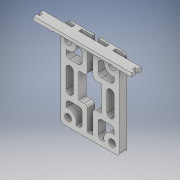
# Autodesk Inventor part: LED Riser
Saved by Autodesk Inventor 2017.3 (Build 213256000, 256)
## iProperties
Created: 2019-07-16
Part Number: LED Riser
Material: Generic
Document SubType Name: Modeling
Designer: LSabe
Density: 1 g/cm^3
Appearance: Default
Author: LSabe
Autodesk Inventor part; units mm, degrees
ref_plane "YZ Plane" through (0, 0, 0) normal (1, 0, 0) x (0, 1, 0)
ref_plane "XZ Plane" through (0, 0, 0) normal (0, 1, 0) x (-1, 0, 0)
ref_plane "XY Plane" through (0, 0, 0) normal (0, 0, 1) x (1, 0, 0)
sketch "Sketch1" plane through (0, 0, 0) normal (0, 0, 1) x (1, 0, 0)
  line L0 (-3.81, -7.6835) -> (45.466, -7.6835)
  line L1 (48.641, -4.5085) -> (48.641, 70.4215)
  line L2 (48.641, 70.4215) -> (-6.985, 70.4215)
  line L3 (-6.985, 70.4215) -> (-6.985, -4.5085)
  arc A0 (45.466, -7.6835) -> (48.641, -4.5085) centre (45.466, -4.5085) ccw
  arc A1 (-6.985, -4.5085) -> (-3.81, -7.6835) centre (-3.81, -4.5085) ccw
  line L4 (31.623, 19.304) -> (31.623, 43.434)
  line L5 (10.033, 43.434) -> (10.033, 19.304)
  line L6 (18.288, -7.6835) -> (23.368, -7.6835)
  line L7 (23.368, 70.4215) -> (18.288, 70.4215)
  arc A2 (-1.905, 55.0979) -> (7.874, 62.738) centre (0, 62.738) ccw
  arc A3 (33.782, 62.738) -> (43.561, 55.0979) centre (41.656, 62.738) ccw
  arc A4 (43.561, 7.6401) -> (34.2249, -2.6035) centre (41.656, 0) ccw
  arc A5 (7.4311, -2.6035) -> (-1.905, 7.6401) centre (0, 0) ccw
  line L8 (34.2249, -2.6035) -> (31.623, -2.6035)
  line L9 (10.033, -2.6035) -> (7.4311, -2.6035)
  line L10 (31.623, 43.434) -> (26.543, 43.434)
  line L11 (15.113, 43.434) -> (10.033, 43.434)
  line L12 (10.033, 19.304) -> (15.113, 19.304)
  line L13 (26.543, 19.304) -> (31.623, 19.304)
  line L14 (23.368, 46.609) -> (23.368, 62.738)
  line L15 (18.288, 62.738) -> (18.288, 46.609)
  line L16 (23.368, -2.6035) -> (23.368, 16.129)
  line L17 (18.288, 16.129) -> (18.288, -2.6035)
  line L18 (18.288, -2.6035) -> (23.368, -2.6035)
  line L19 (28.448, 51.689) -> (28.448, 59.563)
  line L20 (40.386, 48.514) -> (31.623, 48.514)
  line L21 (13.208, 59.563) -> (13.208, 51.689)
  line L22 (10.033, 48.514) -> (1.27, 48.514)
  line L23 (13.208, 11.049) -> (13.208, 0.5715)
  line L24 (1.27, 14.224) -> (10.033, 14.224)
  line L25 (31.623, 14.224) -> (40.386, 14.224)
  line L26 (28.448, 0.5715) -> (28.448, 11.049)
  line L27 (-1.905, 7.6401) -> (-1.905, 11.049)
  line L28 (-1.905, 51.689) -> (-1.905, 55.0979)
  line L29 (43.561, 55.0979) -> (43.561, 51.689)
  line L30 (43.561, 11.049) -> (43.561, 7.6401)
  line L31 (43.561, 22.479) -> (43.561, 40.259)
  line L32 (-1.905, 40.259) -> (-1.905, 22.479)
  line L33 (4.953, 40.259) -> (4.953, 22.479)
  line L34 (36.703, 22.479) -> (36.703, 40.259)
  line L35 (1.27, 43.434) -> (1.778, 43.434)
  line L36 (1.778, 19.304) -> (1.27, 19.304)
  line L37 (39.878, 43.434) -> (40.386, 43.434)
  line L38 (40.386, 19.304) -> (39.878, 19.304)
  arc A6 (10.033, 48.514) -> (13.208, 51.689) centre (10.033, 51.689) ccw
  arc A7 (28.448, 51.689) -> (31.623, 48.514) centre (31.623, 51.689) ccw
  arc A8 (31.623, 14.224) -> (28.448, 11.049) centre (31.623, 11.049) ccw
  arc A9 (13.208, 11.049) -> (10.033, 14.224) centre (10.033, 11.049) ccw
  arc A10 (1.27, 14.224) -> (-1.905, 11.049) centre (1.27, 11.049) ccw
  arc A11 (10.033, -2.6035) -> (13.208, 0.5715) centre (10.033, 0.5715) ccw
  arc A12 (28.448, 0.5715) -> (31.623, -2.6035) centre (31.623, 0.5715) ccw
  arc A13 (43.561, 11.049) -> (40.386, 14.224) centre (40.386, 11.049) ccw
  arc A14 (40.386, 48.514) -> (43.561, 51.689) centre (40.386, 51.689) ccw
  arc A15 (-1.905, 51.689) -> (1.27, 48.514) centre (1.27, 51.689) ccw
  arc A16 (23.368, 46.609) -> (26.543, 43.434) centre (26.543, 46.609) ccw
  arc A17 (15.113, 43.434) -> (18.288, 46.609) centre (15.113, 46.609) ccw
  arc A18 (18.288, 16.129) -> (15.113, 19.304) centre (15.113, 16.129) ccw
  arc A19 (26.543, 19.304) -> (23.368, 16.129) centre (26.543, 16.129) ccw
  arc A20 (36.703, 22.479) -> (39.878, 19.304) centre (39.878, 22.479) ccw
  arc A21 (40.386, 19.304) -> (43.561, 22.479) centre (40.386, 22.479) ccw
  arc A22 (43.561, 40.259) -> (40.386, 43.434) centre (40.386, 40.259) ccw
  arc A23 (39.878, 43.434) -> (36.703, 40.259) centre (39.878, 40.259) ccw
  arc A24 (1.27, 43.434) -> (-1.905, 40.259) centre (1.27, 40.259) ccw
  arc A25 (4.953, 40.259) -> (1.778, 43.434) centre (1.778, 40.259) ccw
  arc A26 (1.778, 19.304) -> (4.953, 22.479) centre (1.778, 22.479) ccw
  arc A27 (-1.905, 22.479) -> (1.27, 19.304) centre (1.27, 22.479) ccw
  line L39 (7.874, 62.738) -> (10.033, 62.738)
  line L40 (18.288, 62.738) -> (23.368, 62.738)
  line L41 (31.623, 62.738) -> (33.782, 62.738)
  arc A28 (13.208, 59.563) -> (10.033, 62.738) centre (10.033, 59.563) ccw
  arc A29 (31.623, 62.738) -> (28.448, 59.563) centre (31.623, 59.563) ccw
  circle A30 centre (0, 62.738) radius 3.302
  circle A31 centre (41.656, 62.738) radius 3.302
  circle A32 centre (0, 0) radius 3.302
  circle A33 centre (41.656, 0) radius 3.302
  point P0 (20.828, 31.369)
  point P1 (23.368, 43.434)
  point P2 (18.288, 43.434)
  point P3 (18.288, 19.304)
  point P4 (23.368, 19.304)
  point P5 (-1.905, 14.224)
  point P6 (43.561, 48.514)
  point P7 (43.561, 14.224)
  point P8 (-1.905, 48.514)
  point P9 (13.208, 65.3415)
  point P10 (28.448, 65.3415)
  point P11 (13.208, -2.6035)
  point P12 (28.448, -2.6035)
  point P13 (28.448, 48.514)
  point P14 (13.208, 48.514)
  point P15 (13.208, 14.224)
  point P16 (28.448, 14.224)
  point P17 (-1.905, 19.304)
  point P18 (43.561, 43.434)
  point P19 (43.561, 19.304)
  point P20 (-1.905, 43.434)
  point P21 (4.953, 43.434)
  point P22 (4.953, 19.304)
  point P23 (36.703, 19.304)
  point P24 (36.703, 43.434)
  point P25 (28.448, 62.738)
  point P26 (13.208, 62.738)
  dimension "d32" = 3.175
  dimension "d37" = 6.604
  dimension "d38" = 6.604
  dimension "d39" = 6.604
  dimension "d40" = 6.604
  constraints: 84 end point, 60 point on circle, 52 point on line, 52 tangent, 34 centre point, 31 parallel, 21 equal radius, 12 horizontal, 9 perpendicular, 4 coincident
  measures "d32" radius of A28
  measures "d37" diameter of A30
  measures "d38" diameter of A31
  measures "d39" diameter of A32
  measures "d40" diameter of A33
extrude "Extrusion1" add sketch "Sketch1" along normal blind 6.985
sketch "Sketch2" plane through (-3.81, -7.6835, 0) normal (0, -1, 0) x (1, 0, 0)
  line L0 (22.098, -3.81) -> (27.178, -3.81)
  line L1 (27.178, -3.81) -> (27.178, 3.81)
  line L2 (27.178, 3.81) -> (22.098, 3.81)
  line L3 (22.098, 3.81) -> (22.098, -3.81)
  line L4 (22.098, -3.81) -> (27.178, 3.81) construction
  line L5 (27.178, -3.81) -> (22.098, 3.81) construction
  point P0 (3.81, 0)
  point P1 (24.638, 0)
  dimension "d28" = 5.08
  dimension "d29" = 7.62
  constraints: 12 end point, 2 midpoint, 2 parallel, 1 horizontal, 1 perpendicular
  measures "d28" distance of L2.end L1.end
  measures "d29" distance of L1.end L0.end
extrude "Extrusion2" cut sketch "Sketch2" against normal blind 115.2525
sketch "Sketch4" plane through (-3.81, 70.4215, 0) normal (0, 1, 0) x (1, 0, 0)
  line L0 (55.626, -6.985) -> (-3.175, -6.985)
  line L1 (26.2255, -6.985) -> (26.2255, 0)
  line L2 (56.3246, -2.2225) -> (-3.8736, -2.2225)
  line L3 (-3.8736, -2.2225) -> (-3.8736, -4.7625)
  line L4 (-3.8736, -4.7625) -> (56.3246, -4.7625)
  line L5 (56.3246, -4.7625) -> (56.3246, -2.2225)
  line L6 (56.3246, -2.2225) -> (-3.8736, -4.7625) construction
  line L7 (-3.8736, -2.2225) -> (56.3246, -4.7625) construction
  point P0 (3.81, 0)
  point P1 (0, -6.985)
  point P2 (26.2255, -3.4925)
  dimension "d41" = 2.54
  constraints: 16 end point, 4 midpoint, 2 parallel, 1 horizontal, 1 perpendicular, 1 vertical
  measures "d41" distance of L3.end L2.end
extrude "Extrusion4" cut sketch "Sketch4" against normal blind 2.794
sketch "Sketch5" plane through (-3.81, 70.4215, 6.985) normal (0, 1, 0) x (1, 0, 0)
  line L0 (-21.717, 2.2225) -> (70.993, 2.2225)
  line L1 (70.993, 2.2225) -> (70.993, -7.3025)
  line L2 (70.993, -7.3025) -> (-21.717, -7.3025)
  line L3 (-21.717, -7.3025) -> (-21.717, 2.2225)
  point P0 (0, 2.2225)
  dimension "d45" = 92.71
  constraints: 8 end point, 2 parallel, 1 horizontal, 1 perpendicular
  measures "d45" distance of L1.end L2.end
extrude "Extrusion5" add sketch "Sketch5" along normal blind 3.556
sketch "Sketch6" plane through (-25.527, 70.4215, 14.2875) normal (0, 1, 0) x (1, 0, 0)
  line L0 (-2.54, 3.4925) -> (2.54, 3.4925)
  line L1 (2.54, 3.4925) -> (2.54, 6.0325)
  line L2 (2.54, 6.0325) -> (-2.54, 6.0325)
  line L3 (-2.54, 6.0325) -> (-2.54, 3.4925)
  line L4 (95.25, 3.4925) -> (90.17, 3.4925)
  line L5 (90.17, 3.4925) -> (90.17, 6.0325)
  line L6 (90.17, 6.0325) -> (95.25, 6.0325)
  line L7 (95.25, 6.0325) -> (95.25, 3.4925)
  point P0 (0, 4.7625)
  point P1 (92.71, 4.7625)
  constraints: 16 end point
extrude "Extrusion6" cut sketch "Sketch6" along normal blind 6.35
sketch "Sketch7" plane through (23.368, 70.4215, 0) normal (0, 1, 0) x (1, 0, 0)
  line L0 (10.4132, -4.7625) -> (16.7632, -4.7625)
  line L1 (-15.4932, -4.7625) -> (-21.8432, -4.7625)
  line L2 (-30.353, 0) -> (-30.353, -6.985) projected
  line L3 (-30.353, -2.2225) -> (-30.353, 0)
  line L4 (25.2501, 0) -> (25.2501, -2.2225)
  line L5 (16.7632, -4.7625) -> (16.7632, -2.2225)
  line L6 (10.4132, -2.2225) -> (10.4132, -4.7625)
  line L7 (-15.4932, -2.2225) -> (-15.4932, -4.7625)
  line L8 (-21.8432, -4.7625) -> (-21.8432, -2.2225)
  line L9 (-21.8432, -2.2225) -> (-30.353, -2.2225)
  line L10 (25.2501, -2.2225) -> (16.7632, -2.2225)
  line L11 (-5.08, -2.2225) -> (-5.08, 0)
  line L12 (0, -2.2225) -> (0, 0)
  line L13 (10.4132, -2.2225) -> (0, -2.2225)
  line L14 (-5.08, -2.2225) -> (-15.4932, -2.2225)
  line L15 (-30.353, 0) -> (-5.08, 0)
  line L16 (0, 0) -> (25.2501, 0)
  point P0 (-23.368, 0)
  constraints: 32 end point, 10 parallel, 5 horizontal, 5 perpendicular, 2 vertical
extrude "Extrusion7" add sketch "Sketch7" along normal up to surface (3.556 mm away)
fillet "Fillet1" radius 3.175 2 edges at (-6.985, 73.9775, 1.1113) (48.6181, 73.9775, 1.1113)
sketch "Sketch8" plane through (-25.527, 70.4215, 14.2875) normal (0, 0, 1) x (1, 0, 0)
  line L0 (74.168, 0) -> (18.542, 0) projected
  line L1 (18.542, 0) -> (74.168, 0)
  line L2 (74.168, 0) -> (74.168, 0.635)
  line L3 (74.168, 0.635) -> (18.542, 0.635)
  line L4 (18.542, 0.635) -> (18.542, 0)
  point P0 (25.527, -70.4215)
  dimension "d58" = 55.626
  dimension "d59" = 0.635
  constraints: 8 end point, 2 parallel, 1 horizontal, 1 perpendicular
  measures "d58" distance of L3.end L2.end
  measures "d59" distance of L2.end L1.end
extrude "Extrusion8" cut sketch "Sketch8" against normal up to surface (7.3025 mm away)
chamfer "Chamfer1" distance 0.635 angle 45 1 edges at (-6.985, 70.4215, 10.6363)
chamfer "Chamfer2" distance 0.635 angle 45 1 edges at (48.641, 70.4215, 10.6363)
sketch "Sketch9" plane through (23.368, 67.6275, 2.2225) normal (0, 0, 1) x (1, 0, 0)
  arc A0 (25.2501, 3.175) -> (22.0751, 6.35) centre (22.0751, 3.175) ccw projected
  line L0 (22.0751, 6.35) -> (16.7632, 6.35) projected
  line L1 (16.7632, 2.794) -> (16.7632, 6.35) projected
  line L2 (10.4132, 2.794) -> (16.7632, 2.794) projected
  line L3 (10.4132, 2.794) -> (10.4132, 6.35) projected
  line L4 (10.4132, 6.35) -> (0, 6.35) projected
  line L5 (0, 0) -> (0, 6.35) projected
  line L6 (0, 0) -> (25.273, 0) projected
  line L7 (25.273, 2.794) -> (25.273, 0) projected
  line L8 (25.2501, 2.794) -> (25.273, 2.794) projected
  line L9 (25.2501, 2.794) -> (25.2501, 3.175) projected
  arc A1 (-27.178, 6.35) -> (-30.353, 3.175) centre (-27.178, 3.175) ccw projected
  line L10 (-30.353, 0) -> (-30.353, 3.175) projected
  line L11 (-30.353, 0) -> (-5.08, 0) projected
  line L12 (-5.08, 6.35) -> (-5.08, 0) projected
  line L13 (-5.08, 6.35) -> (-15.4932, 6.35) projected
  line L14 (-15.4932, 2.794) -> (-15.4932, 6.35) projected
  line L15 (-21.8432, 2.794) -> (-15.4932, 2.794) projected
  line L16 (-21.8432, 2.794) -> (-21.8432, 6.35) projected
  line L17 (-21.8432, 6.35) -> (-27.178, 6.35) projected
  point P0 (-23.368, -67.6275)
extrude "Extrusion9" cut sketch "Sketch9" along normal blind 2.794 and the other way blind 0.254
sketch "Sketch10" plane through (23.368, 67.6275, 4.7625) normal (0, 0, -1) x (-1, 0, 0)
  line L0 (0, 6.35) -> (0, 0) projected
  line L1 (0, 0) -> (5.08, 0) projected
  line L2 (5.08, 0) -> (5.08, 6.35) projected
  line L3 (0, 6.35) -> (5.08, 6.35) projected
  point P0 (23.368, -67.6275)
extrude "Extrusion10" cut sketch "Sketch10" against normal blind 0.254
sketch "Sketch11" plane through (40.1312, 70.4215, 5.0165) normal (1, 0, 0) x (0, 0, -1)
  point P0 (5.0165, -70.4215)
sketch "Sketch12" plane through (67.183, 70.4215, 4.7625) normal (0, 0, -1) x (-1, 0, 0)
  line L0 (18.5649, 0) -> (0, 0) projected
  line L1 (18.5649, 0) -> (18.5649, 0.381) projected
  arc A0 (21.7399, 3.556) -> (18.5649, 0.381) centre (21.7399, 0.381) ccw projected
  line L2 (0, 3.556) -> (21.7399, 3.556) projected
  line L3 (0, 0) -> (0, 3.556) projected
  arc A1 (74.168, 0.381) -> (70.993, 3.556) centre (70.993, 0.381) ccw projected
  line L4 (74.168, 0.381) -> (74.168, 0) projected
  line L5 (92.71, 0) -> (74.168, 0) projected
  line L6 (92.71, 0) -> (92.71, 3.556) projected
  line L7 (70.993, 3.556) -> (92.71, 3.556) projected
  point P0 (67.183, -70.4215)
extrude "Extrusion11" cut sketch "Sketch12" against normal blind 0.254
body "Solid1"
